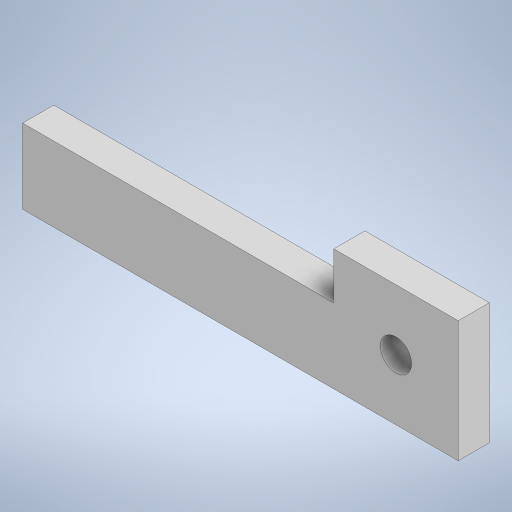
# Autodesk Inventor part: Touchscreen mount v02
Saved by Autodesk Inventor 2023 (Build 270158000, 158)
## iProperties
Created: 2024-06-28
Part Number: Touchscreen mount v02
Material: Generic
Document SubType Name: Modeling
Designer: Akramilab
Density: 1 g/cm^3
Appearance: Default
Author: Akramilab
Autodesk Inventor part; units mm, degrees
ref_plane "YZ Plane" through (0, 0, 0) normal (1, 0, 0) x (0, 1, 0)
ref_plane "XZ Plane" through (0, 0, 0) normal (0, 1, 0) x (-1, 0, 0)
ref_plane "XY Plane" through (0, 0, 0) normal (0, 0, 1) x (1, 0, 0)
sketch "Sketch1" plane through (0, 0, 0) normal (0, 0, 1) x (1, 0, 0)
  line L0 (0, 0) -> (70, 0)
  line L1 (70, 0) -> (70, -12)
  line L2 (70, -12) -> (0, -12)
  line L3 (0, -12) -> (0, 0)
  line L4 (70, 0) -> (50, 0)
  line L5 (50, 0) -> (50, 7.5)
  line L6 (50, 7.5) -> (70, 7.5)
  line L7 (70, 7.5) -> (70, 0)
  circle A0 centre (60, -2.25) radius 2.5
  point P0 (0, -6)
  point P1 (70, -6)
  point P2 (35, 0)
  point P3 (50, 0)
  dimension "d0" = 70
  dimension "d1" = 12
  dimension "d11" = 20
  dimension "d12" = 7.5
  dimension "d15" = 9.75
  dimension "d16" = 10
  dimension "d17" = 5
  constraints: 16 end point, 4 parallel, 3 midpoint, 2 horizontal, 2 perpendicular, 1 centre point, 1 coincident
  measures "d0" distance of L1.end L2.end
  measures "d1" distance of L0.end L1.end
  measures "d11" distance of L5.end L6.end
  measures "d12" distance of L4.end L5.end
  measures "d15" distance from line of L2 point (60, -2.25)
  measures "d16" distance from line of L1 point (60, -2.25)
  measures "d17" diameter of A0
extrude "Extrusion2" add sketch "Sketch1" along normal blind 5 contours L0 A0 L1 L2 L3 | L5 L6 L7 L0 A0
equation "\"d15\" = 0.5 * d1 + 0.5 * d12"
equation "\"d16\" = 0.5 * d11"
body "Solid2"
